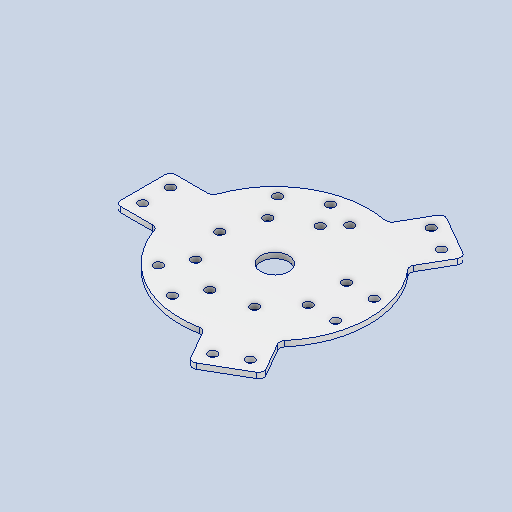
# Autodesk Inventor part: hand-grab-v1-MDF-air-Base
Saved by Autodesk Inventor 2025.2 (Build 292293000, 293)
## iProperties
Created: 2024-10-07
Part Number: hand-grab-v1-MDF-air-Base
Material: アルミニウム 6061
Document SubType Name: Modeling
Designer: haruy
Density: 2.7 g/cm^3
Appearance: アルミニウム - フラット
Author: haruy
Autodesk Inventor part; units mm, degrees
ref_plane "YZ Plane" through (0, 0, 0) normal (1, 0, 0) x (0, 1, 0)
ref_plane "XZ Plane" through (0, 0, 0) normal (0, 1, 0) x (-1, 0, 0)
ref_plane "XY Plane" through (0, 0, 0) normal (0, 0, 1) x (1, 0, 0)
derived "hand-grab-v1-Sketch-Base.ipt"
sketch "スケッチ1" plane through (400, 0, 0) normal (1, 0, 0) x (0, 1, 0)
  circle A0 centre (0, 0) radius 120
  circle A1 centre (-109.5522, 63.25) radius 6.5
  line L0 (0, 0) -> (-109.5522, 63.25)
  line L1 (0, 0) -> (0, 120)
  line L2 (246.0862, 200) -> (-251.4603, 200)
  circle A2 centre (145, 60) radius 254.573
  circle A3 centre (-67.6203, 200) radius 6.5
  line L3 (0, 0) -> (-120, 0)
  line L4 (249, 9.15) -> (187, 9.15)
  line L5 (187, 9.15) -> (187, -9.15)
  line L6 (187, -9.15) -> (249, -9.15)
  line L7 (249, -9.15) -> (249, 9.15)
  line L8 (187, 5.15) -> (179, 5.15)
  line L9 (179, 5.15) -> (179, -4.85)
  line L10 (179, -4.85) -> (187, -4.85)
  line L11 (187, -4.85) -> (187, 5.15)
  line L12 (179, 3.15) -> (174, 3.15)
  line L13 (174, 3.15) -> (174, -2.85)
  line L14 (174, -2.85) -> (179, -2.85)
  line L15 (179, -2.85) -> (179, 3.15)
  line L16 (174, 2.65) -> (159, 2.65)
  line L17 (159, 2.65) -> (159, -2.35)
  line L18 (159, -2.35) -> (174, -2.35)
  line L19 (174, -2.35) -> (174, 2.65)
  line L20 (187, 34.15) -> (184, 34.15)
  line L21 (184, 34.15) -> (184, -43.5182)
  line L22 (184, -43.5182) -> (187, -43.5182)
  line L23 (187, -43.5182) -> (187, 34.15)
  circle A4 centre (150, 65) radius 4
  circle A5 centre (150, 65) radius 14
  line L24 (187, 34.15) -> (192, 34.15)
  line L25 (192, 34.15) -> (192, 14.15)
  line L26 (192, 14.15) -> (187, 14.15)
  line L27 (187, 14.15) -> (187, 34.15)
  line L28 (184, 34.15) -> (147.5804, 61.8148)
  line L29 (151.3533, 68.7641) -> (192, 54.15)
  line L30 (192, 54.15) -> (192, 34.15)
  line L31 (239.3868, 130) -> (-239.3868, 130)
  circle A6 centre (-109.5522, 63.25) radius 4
  circle A7 centre (150, 65) radius 9
  line L32 (-106.0881, 61.25) -> (-113.0163, 65.25)
  line L33 (170, 36) -> (155, 36)
  circle A8 centre (155, 36) radius 5
  circle A9 centre (155, 36) radius 9
  circle A10 centre (-90.698, 156.1969) radius 6.5
  circle A11 centre (170, 36) radius 5
  line L34 (150, 65) -> (170, 36)
  circle A12 centre (170, 36) radius 9
  circle A13 centre (150, 65) radius 44.2278
  line L35 (150, 65) -> (155, 36)
  line L36 (150, 65) -> (-109.5522, 63.25)
  line L37 (-90.698, 156.1969) -> (150, 65)
  line L38 (150, 65) -> (157.5146, 21.4152)
  circle A14 centre (150, 65) radius 35.2278
  circle A15 centre (155.9855, 30.2844) radius 9
  line L39 (168.0777, 21.2844) -> (136, 21.2844)
  line L40 (175, 3.15) -> (175, -2.85)
  point P0 (-60, 0)
sketch "スケッチ2" plane through (0, 400, 0) normal (0, 1, 0) x (-1, 0, 0)
  circle A0 centre (0, 0) radius 120
  line L0 (0, 0) -> (-331.4625, 0) construction
  line L1 (67.5, -116.9134) -> (-135, 0)
  circle A1 centre (0, 0) radius 5.1
  line L2 (0, 0) -> (67.5, 116.9134) construction
  line L3 (0, 0) -> (67.5, -116.9134) construction
  line L4 (0, 0) -> (-135, 0)
  line L5 (17.0359, 37.507) -> (12.0359, 28.8468) construction
  line L6 (12.0359, 28.8468) -> (15.5, 26.8468) construction
  line L7 (15.5, 26.8468) -> (20.5, 35.507) construction
  line L8 (20.5, 35.507) -> (17.0359, 37.507)
  line L9 (20.5, 35.507) -> (15.5, 26.8468) construction
  line L10 (15.5, 26.8468) -> (18.9641, 24.8468) construction
  line L11 (18.9641, 24.8468) -> (23.9641, 33.507) construction
  line L12 (23.9641, 33.507) -> (20.5, 35.507)
  line L13 (14.5359, 33.1769) -> (21.4641, 29.1769) construction
  circle A2 centre (0, 0) radius 2.6 construction
  line L14 (16.8194, 37.632) -> (10.3194, 26.3737) construction
  line L15 (10.3194, 26.3737) -> (5.9893, 28.8737) construction
  line L16 (5.9893, 28.8737) -> (12.4893, 40.132) construction
  line L17 (12.4893, 40.132) -> (16.8194, 37.632)
  line L18 (28.5107, 30.882) -> (24.1806, 33.382)
  line L19 (22.0107, 19.6237) -> (28.5107, 30.882) construction
  line L20 (24.1806, 33.382) -> (17.6806, 22.1237) construction
  line L21 (17.6806, 22.1237) -> (22.0107, 19.6237) construction
  circle A3 centre (0, 0) radius 28.3207 construction
  line L22 (-41, 9.25) -> (-41, 4.25)
  line L23 (-41, 4.25) -> (-28, 4.25) construction
  line L24 (-28, 9.25) -> (-41, 9.25) construction
  line L25 (-28, 4.25) -> (-28, 9.25)
  line L26 (-41, -4.25) -> (-28, -4.25) construction
  line L27 (-41, -9.25) -> (-41, -4.25)
  line L28 (-28, -9.25) -> (-41, -9.25) construction
  line L29 (-28, -4.25) -> (-28, -9.25)
  line L30 (12.4893, -40.132) -> (16.8194, -37.632)
  line L31 (16.8194, -37.632) -> (10.3194, -26.3737) construction
  line L32 (5.9893, -28.8737) -> (12.4893, -40.132) construction
  line L33 (10.3194, -26.3737) -> (5.9893, -28.8737) construction
  line L34 (24.1806, -33.382) -> (17.6806, -22.1237) construction
  line L35 (28.5107, -30.882) -> (24.1806, -33.382)
  line L36 (22.0107, -19.6237) -> (28.5107, -30.882) construction
  line L37 (17.6806, -22.1237) -> (22.0107, -19.6237) construction
  line L38 (5.9893, 28.8737) -> (5.373, 27.8064)
  line L39 (22.0107, 19.6237) -> (21.3945, 18.5564) construction
  line L40 (-28, 9.25) -> (-26.7675, 9.25)
  line L41 (-28, -9.25) -> (-26.7675, -9.25)
  line L42 (5.9893, -28.8737) -> (2.1934, -22.2991)
  line L43 (22.0107, -19.6237) -> (21.3945, -18.5564) construction
  line L44 (13.6109, 31.5748) -> (3.6109, 14.2543) construction
  line L45 (3.6109, 14.2543) -> (-1.5853, 17.2543) construction
  line L46 (-1.5853, 17.2543) -> (8.4147, 34.5748) construction
  line L47 (8.4147, 34.5748) -> (13.6109, 31.5748)
  circle A4 centre (3.5128, 20.0844) radius 1.6
  circle A5 centre (8.5128, 28.7446) radius 1.6
  circle A6 centre (20.6372, 21.7446) radius 1.6
  circle A7 centre (15.6372, 13.0844) radius 1.6
  circle A8 centre (-29.15, 7) radius 1.6
  circle A9 centre (-19.15, 7) radius 1.6
  circle A10 centre (-19.15, -7) radius 1.6
  circle A11 centre (-29.15, -7) radius 1.6
  circle A12 centre (8.5128, -28.7446) radius 1.6
  circle A13 centre (3.5128, -20.0844) radius 1.6
  circle A14 centre (15.6372, -13.0844) radius 1.6
  circle A15 centre (20.6372, -21.7446) radius 1.6
  line L48 (1.0128, 15.7543) -> (13.6109, 31.5748) construction
  circle A16 centre (0, 0) radius 34.3835
  line L49 (-8, 47) -> (-188, 47) construction
  line L50 (-188, 47) -> (-188, 32)
  line L51 (-188, 32) -> (-8, 32) construction
  line L52 (-8, 32) -> (-8, 47) construction
  circle A17 centre (-18, 39.5) radius 1.5 construction
  circle A18 centre (-28, 39.5) radius 1.5 construction
  line L53 (-34.3835, 47) -> (-34.3835, 0) construction
  line L54 (-8, 47) -> (19.3201, 28.4422) construction
  line L55 (-8, -47) -> (-188, -47) construction
  line L56 (-188, -32) -> (-8, -32) construction
  circle A19 centre (-18, -39.5) radius 1.5 construction
  circle A20 centre (-28, -39.5) radius 1.5 construction
  line L57 (-34.3835, -47) -> (-34.3835, 0) construction
  line L58 (-8, -47) -> (19.3201, -28.4422) construction
  line L59 (0, 0) -> (-17.1917, 29.777)
  line L60 (-15.3397, 46.5692) -> (-32.6603, 36.5692)
  line L61 (-32.6603, 36.5692) -> (-27.6603, 27.909)
  line L62 (-27.6603, 27.909) -> (-10.3397, 37.909)
  line L63 (-10.3397, 37.909) -> (-15.3397, 46.5692)
  circle A21 centre (-17.1699, 39.7391) radius 1.6
  circle A22 centre (-25.8301, 34.7391) radius 1.6
  circle A23 centre (-25.8301, -34.7391) radius 1.6
  circle A24 centre (-17.1699, -39.7391) radius 1.6
  circle A25 centre (43, -5) radius 1.6
  circle A26 centre (43, 5) radius 1.6
  circle A27 centre (0, 0) radius 193.5
  line L64 (-192.8647, 15.6665) -> (82.8647, 174.859)
  line L65 (0, 0) -> (-60, 103.923)
  line L66 (0, 0) -> (0, 193.5)
  line L67 (48.9711, 5.1795) -> (-52.5289, 180.9826)
  line L68 (-52.5289, 180.9826) -> (-69.8494, 170.9826)
  line L69 (-69.8494, 170.9826) -> (31.6506, -4.8205)
  line L70 (31.6506, -4.8205) -> (48.9711, 5.1795)
  circle A28 centre (-30.6042, 118.008) radius 1.5
  circle A29 centre (-55.274, 170.7375) radius 1.5
  circle A30 centre (-10, 17.3205) radius 1.6
  circle A31 centre (0, 0) radius 10 construction
  circle A32 centre (35.3109, 8.8397) radius 1.5
  circle A33 centre (25.3109, 26.1603) radius 1.5
  line L71 (48.9711, 5.1795) -> (22.0795, -10.3464)
  line L72 (28.9711, 39.8205) -> (-4.4157, 20.5446)
  line L73 (-28.9711, -39.8205) -> (-130.4711, 135.9826)
  line L74 (-11.6506, -29.8205) -> (-28.9711, -39.8205)
  circle A34 centre (-25.3109, -26.1603) radius 1.5
  circle A35 centre (-35.3109, -8.8397) radius 1.5
  line L75 (-28.9711, -39.8205) -> (-2.0795, -24.2946)
  line L76 (-48.9711, -5.1795) -> (-15.5843, 14.0964)
  line L77 (0, 0) -> (-17.1917, -29.777)
  line L78 (0.6292, -11.9103) -> (-10.6292, -5.4103) construction
  line L79 (-10.6292, -5.4103) -> (-19.6292, -20.9987) construction
  line L80 (-19.6292, -20.9987) -> (-8.3708, -27.4987) construction
  line L81 (-8.3708, -27.4987) -> (0.6292, -11.9103) construction
  circle A36 centre (0, 0) radius 28
  circle A37 centre (0, 0) radius 38 construction
  circle A38 centre (0, 0) radius 12.5 construction
  circle A39 centre (-10, -17.3205) radius 1.6
  circle A40 centre (20, 0) radius 1.6
  circle A41 centre (-1.5877, -25.75) radius 3
  circle A42 centre (-1.5877, -25.75) radius 1.6
  line L82 (-10.3397, 37.909) -> (-7.7883, 33.4898)
  line L83 (-27.6603, 27.909) -> (-25.1088, 23.4898)
  line L84 (-10.3397, -37.909) -> (-7.7883, -33.4898)
  line L85 (-15.3397, -46.5692) -> (-10.3397, -37.909)
  line L86 (-32.6603, -36.5692) -> (-15.3397, -46.5692)
  circle A43 centre (-17.1699, -39.7391) radius 1.6
  circle A44 centre (-25.8301, -34.7391) radius 1.6
  line L87 (-27.6603, -27.909) -> (-32.6603, -36.5692)
  line L88 (-27.6603, -27.909) -> (-25.1088, -23.4898)
  line L89 (38, 10) -> (32.8972, 10)
  line L90 (48, 10) -> (38, 10)
  line L91 (48, -10) -> (48, 10)
  circle A45 centre (43, 5) radius 1.6
  circle A46 centre (43, -5) radius 1.6
  line L92 (38, -10) -> (48, -10)
  line L93 (38, -10) -> (32.8972, -10)
  point P0 (19.3201, -28.4422)
  point P1 (-15.1292, -13.2045)
  point P2 (-24, 41.5692)
  point P3 (-24, -41.5692)
  point P4 (48, 0)
  dimension "d3" = 3
  dimension "d4" = 3
  dimension "d5" = 10
  dimension "d6" = 10
  dimension "d7" = 7.5
  dimension "d8" = 7.5
  dimension "d10" = 60
  dimension "d12" = 10
  dimension "d13" = 10
  dimension "d14" = 10
  dimension "d15" = 3.2
  dimension "d17" = 5
  dimension "d18" = 5
  dimension "d21" = 360
  dimension "d25" = 387
  dimension "d26" = 110
  dimension "d27" = 60
  dimension "d28" = 20
  dimension "d30" = 73
  dimension "d31" = 3
  dimension "d32" = 3
  dimension "d33" = 7.5
  dimension "d34" = 7.5
  dimension "d35" = 7.5
  dimension "d36" = 7.5
  dimension "d37" = 3.2
  dimension "d38" = 20
  dimension "d44" = 20
  dimension "d45" = 3
  dimension "d46" = 3
  dimension "d47" = 10
  dimension "d48" = 10
  dimension "d49" = 10
  dimension "d50" = 20
  dimension "d52" = 10
  dimension "d53" = 120
  dimension "d54" = 13
  dimension "d55" = 18
  dimension "d56" = 6.5
  dimension "d57" = 56
  dimension "d58" = 10
  dimension "d59" = 25
  dimension "d60" = 25
  dimension "d61" = 20
  dimension "d64" = 360
  dimension "d66" = 6
  dimension "d67" = 5
  dimension "d68" = 5
  dimension "d69" = 3.2
  dimension "d72" = 360
  measures "d3" diameter of A17
  measures "d4" diameter of A18
  measures "d5" distance from line of A17.centre L52
  measures "d6" distance of A18.centre A17.centre
  measures "d7" distance from line of A17.centre L49
  measures "d8" distance from line of L49 A18.centre
  measures "d12" distance between parallel lines of L60 L62
  measures "d13" distance between parallel lines of L63 L59
  measures "d14" distance between parallel lines of L59 L61
  measures "d15" diameter of A21
  measures "d17" distance from line of L59 A21.centre
  measures "d18" distance from line of A21.centre L60
  measures "d25" diameter of A27
  measures "d26" distance from line of L64 A3.centre
  measures "d28" distance of L68.end L67.end
  measures "d30" distance between parallel lines of L64 L68
  measures "d31" diameter of A28
  measures "d32" diameter of A29
  measures "d33" distance from line of A28.centre L64
  measures "d34" distance from line of A28.centre L69
  measures "d35" distance from line of A29.centre L68
  measures "d36" distance from line of A29.centre L67
  measures "d37" diameter of A30
  measures "d38" diameter of A31
  measures "d44" distance from line of L70 point (0, 0)
  measures "d45" diameter of A32
  measures "d46" diameter of A33
  measures "d47" distance from line of A32.centre L70
  measures "d48" distance from line of L67 A33.centre
  measures "d49" distance from line of L67 A32.centre
  measures "d50" distance of A33.centre A32.centre
  measures "d52" distance from line of L72 A33.centre
  measures "d54" distance from line of point (-15.129, -13.204) L81
  measures "d55" distance between parallel lines of L78 L80
  measures "d56" distance between parallel lines of L77 L81
  measures "d57" diameter of A36
  measures "d58" radial gap between concentric circles of A36 A37
  measures "d59" diameter of A38
  measures "d60" distance from line of L69 L4.start
  measures "d61" distance of point (0, 0) A30.centre
  measures "d66" diameter of A41
  measures "d67" distance from line of L81 A41.centre
  measures "d68" distance from line of A41.centre L42
  measures "d69" diameter of A42
ref_plane "作業平面1" through (400, 0, 0) normal (1, 0, 0) x (0, 1, 0)
ref_plane "作業平面2" through (0, 400, 0) normal (0, 1, 0) x (-1, 0, 0)
extrude "押し出し1" add sketch "スケッチ2" against normal blind 2 contours L66 A36 L59 A16 | A16 L69 L72 A5 A36 L66 | L90 L91 L67 | L67 L91 L70 A16 L89 A32 L90 | A16 L72 L69 | A16 L65 L62 L82 | A36 L72 L66 | L66 A1 L59 A30 A36 | A16 L70 L69 A36 L72 | L65 L62 L61 L60 | L60 L63 L62 L65 | L69 A36 L72 A5 | L59 A36 L76 A8 A16 | A16 L83 L62 L65 | L72 A36 L69 A41 L75 L77 A39 A1 L66 | L59 A30 A1 L4 A36 | L91 L92 L93 A16 L70 | A32 L89 | A16 L76 A8 A36 L4 | L4 A36 L77 A16 | L87 L88 A34 A16 L74 L86 L73 | L73 L86 L87 | A36 L69 | A16 L74 L75 A36 A41 L71 L70 | L4 A1 L77 A39 A36 | L69 L71 A36 | A36 L75 L74 A16 L77 | A34 L88 | L74 A16 L84 L85 L86 | A39 L77 | L77 A39 | L75 A41 A36 | A41 A36 | A36 A41 picked at (35.7858, 8.8006) picked at (-25.2781, -26.6201)
sketch "スケッチ4" plane through (0, 398, 0) normal (0, -1, 0) x (1, 0, 0)
  arc A0 (25.1088, -23.4898) -> (25.1088, 23.4898) centre (0, 0) ccw projected
  circle A1 centre (0, 0) radius 5.1 projected
  circle A2 centre (19.15, 7) radius 1.6 projected
  circle A3 centre (29.15, -7) radius 1.6 projected
  circle A4 centre (-8.5128, -28.7446) radius 1.6 projected
  circle A5 centre (-20.6372, -21.7446) radius 1.6 projected
  circle A6 centre (29.15, 7) radius 1.6 projected
  circle A7 centre (-15.6372, -13.0844) radius 1.6 projected
  circle A8 centre (-3.5128, -20.0844) radius 1.6 projected
  circle A9 centre (19.15, -7) radius 1.6 projected
  circle A10 centre (-15.6372, 13.0844) radius 1.6 projected
  circle A11 centre (-3.5128, 20.0844) radius 1.6 projected
  circle A12 centre (-8.5128, 28.7446) radius 1.6 projected
  circle A13 centre (-20.6372, 21.7446) radius 1.6 projected
  circle A14 centre (10, 17.3205) radius 1.6 projected
  line L0 (15.3397, 46.5692) -> (7.7883, 33.4898) projected
  arc A15 (7.7883, 33.4898) -> (-32.8972, 10) centre (0, 0) ccw projected
  line L1 (-32.8972, 10) -> (-48, 10) projected
  line L2 (-48, 10) -> (-48, -10) projected
  line L3 (-48, -10) -> (-32.8972, -10) projected
  arc A16 (-32.8972, -10) -> (7.7883, -33.4898) centre (0, 0) ccw projected
  line L4 (7.7883, -33.4898) -> (15.3397, -46.5692) projected
  line L5 (15.3397, -46.5692) -> (32.6603, -36.5692) projected
  line L6 (32.6603, -36.5692) -> (25.1088, -23.4898) projected
  line L7 (25.1088, 23.4898) -> (32.6603, 36.5692) projected
  line L8 (32.6603, 36.5692) -> (15.3397, 46.5692) projected
fillet "フィレット2" radius 2 12 edges at (7.7883, 399, -33.4898) (15.3397, 399, -46.5692) (32.6603, 399, -36.5692) (25.1088, 399, -23.4898) (25.1088, 399, 23.4898) (32.6603, 399, 36.5692) (15.3397, 399, 46.5692) (7.7883, 399, 33.4898) (-32.8972, 399, 10) (-48, 399, 10) (-32.8972, 399, -10) (-48, 399, -10)
equation "\"d8\" = d7"
